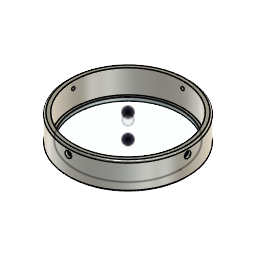
Experimental Hold v13 (Autodesk Fusion 360 design; units mm, degrees)
Autodesk Fusion 360 part; units mm, degrees
sketch "Sketch1" plane through (0, 0, 0) normal (0, 0, 1) x (1, 0, 0)
  circle A0 centre (0, 0) radius 35.5
  circle A1 centre (0, 0) radius 32.5
  dimension "d2" = 71
  dimension "d3" = 65
  measures "d2" diameter of A0
  measures "d3" diameter of A1
extrude "Extrude1" add sketch "Sketch1" along normal blind 14
sketch "Sketch2" plane through (0, 0, 0) normal (0, 0, 1) x (1, 0, 0)
  circle A0 centre (0, 0) radius 31
  dimension "d8" = 62
  constraint coincident A0.centre origin
  measures "d8" diameter of A0
sketch "Sketch3" plane through (0, 0, 0) normal (0, 0, 1) x (1, 0, 0)
  circle A0 centre (0, 0) radius 32.5
  circle A1 centre (0, 0) radius 31.0483
  constraint coincident A0.centre A1.centre
extrude "Extrude3" add sketch "Sketch3" sketch "Sketch1" against normal blind 2.15 of sketch 2
fillet "Fillet1" radius 1 1 edges at (-33.0976, 12.8373, -2.15)
sketch "Sketch4" plane through (0, 0, 0) normal (0, 1, 0) x (1, 0, 0)
  line L0 (-35.5, -14) -> (35.5, -14)
  line L1 (0, -14) -> (0, -11)
  circle A0 centre (0, -10) radius 1
  dimension "d13" = 3
  dimension "d14" = 2
  constraint midpoint L0 L1.start
  constraint perpendicular L0 L1
  constraint coincident L1.end A0
  measures "d13" distance of L1.start L1.end
  measures "d14" diameter of A0
extrude "Extrude4" cut sketch "Sketch4" along normal through all and the other way through all
sketch "Sketch5" plane through (0, 0, 0) normal (1, 0, 0) x (0, 1, 0)
  line L0 (0, 14) -> (0, 11)
  circle A0 centre (0, 10) radius 1
  point P0 (0, 14)
  dimension "d16" = 3
  dimension "d17" = 2
  constraint coincident P0 L0.start
  constraint vertical L0
  constraint coincident L0.end A0
  measures "d16" distance of P0 L0.end
  measures "d17" diameter of A0
extrude "Extrude5" cut sketch "Sketch5" along normal through all and the other way through all
ref_plane "WorkPlane1" through (0, 35.5, 0) normal (0, 1, 0) x (0, 0, 1)
sketch "Sketch6" plane through (0, 35.5, 0) normal (0, 1, 0) x (1, 0, 0)
  circle A0 centre (0, -10) radius 1.9
  dimension "d24" = 3.8
  measures "d24" diameter of A0
extrude "Extrude6" cut sketch "Sketch6" against normal blind 1.5
ref_plane "WorkPlane2" through (0, -35.5, 0) normal (0, 1, 0) x (0, 0, 1)
sketch "Sketch7" plane through (0, -35.5, 0) normal (0, 1, 0) x (1, 0, 0)
  circle A0 centre (0, -10) radius 1.9
  circle A1 centre (0, -10) radius 1
  dimension "d28" = 3.8
  constraint concentric A0 A1
  measures "d28" diameter of A0
extrude "Extrude7" cut sketch "Sketch7" along normal blind 1.5
ref_plane "WorkPlane3" through (-35.5, 0, 0) normal (1, 0, 0) x (0, 1, 0)
sketch "Sketch8" plane through (-35.5, 0, 0) normal (1, 0, 0) x (0, 1, 0)
  circle A0 centre (0, 9.9) radius 1.9
  dimension "d32" = 3.8
  measures "d32" diameter of A0
extrude "Extrude8" cut sketch "Sketch8" along normal blind 1.5
ref_plane "WorkPlane4" through (35.5, 0, 0) normal (1, 0, 0) x (0, 1, 0)
sketch "Sketch9" plane through (35.5, 0, 0) normal (1, 0, 0) x (0, 1, 0)
  circle A0 centre (0, 9.9) radius 1.9
  circle A1 centre (0, 9.9) radius 1.9
  dimension "d36" = 3.8
  constraint concentric A0 A1
  measures "d36" diameter of A0
extrude "Extrude9" cut sketch "Sketch9" against normal blind 1.5
fillet "Fillet3" radius 1 1 edges at (-33.0976, -12.8373, 14)
